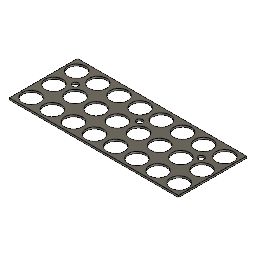
3x8_pcb_mask (Autodesk Fusion 360 design; units mm, degrees)
Autodesk Fusion 360 part; units mm, degrees
sketch "3x8-Edge_Cuts" plane through (0, 0, 0) normal (0, 0, 1) x (1, 0, 0)
  line L0 (17, -29.5) -> (17, -100.6)
  line L1 (17, -100.6) -> (193, -100.6)
  line L2 (193, -29.5) -> (17, -29.5)
  line L3 (193, -100.6) -> (193, -29.5)
sketch "3x8-User_Comments" plane through (0, 0, 0) normal (0, 0, 1) x (1, 0, 0)
  circle A0 centre (105.98, -53.92) radius 3
  circle A1 centre (39.54, -54.16) radius 3
  circle A2 centre (170.85, -54.72) radius 3
sketch "3x8-User_Drawings" plane through (0, 0, 0) normal (0, 0, 1) x (1, 0, 0)
  circle A0 centre (138.077, -65.15) radius 9
  circle A1 centre (28.0768, -41.45) radius 9
  circle A2 centre (138.077, -88.85) radius 9
  circle A3 centre (72.0768, -88.85) radius 9
  circle A4 centre (116.077, -88.85) radius 9
  circle A5 centre (50.0768, -41.45) radius 9
  circle A6 centre (94.0768, -41.45) radius 9
  circle A7 centre (160.077, -88.85) radius 9
  circle A8 centre (72.0768, -41.45) radius 9
  circle A9 centre (138.077, -41.45) radius 9
  circle A10 centre (50.0768, -65.15) radius 9
  circle A11 centre (28.0768, -88.85) radius 9
  circle A12 centre (116.077, -41.45) radius 9
  circle A13 centre (94.0768, -88.85) radius 9
  circle A14 centre (28.0768, -65.15) radius 9
  circle A15 centre (116.077, -65.15) radius 9
  circle A16 centre (160.077, -41.45) radius 9
  circle A17 centre (160.077, -65.15) radius 9
  circle A18 centre (50.0768, -88.85) radius 9
  circle A19 centre (94.0768, -65.15) radius 9
  circle A20 centre (182.077, -65.15) radius 9
  circle A21 centre (182.077, -41.45) radius 9
  circle A22 centre (182.077, -88.85) radius 9
  circle A23 centre (72.0768, -65.15) radius 9
extrude "Extrude1" add sketch "3x8-Edge_Cuts" along normal blind 2
extrude "Extrude2" cut sketch "3x8-User_Drawings" sketch "3x8-User_Comments" along normal blind 2 of sketch 2
